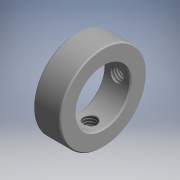
# Autodesk Inventor part: SCCJ10-5_b
Saved by Autodesk Inventor 2017.3 (Build 213256000, 256)
## iProperties
Part Number: SCCJ10-5_b
Material: Generic
Catalog Web Link: www.cadenas.de
Description: SCCJ, PSCCJ, SSCCJ_body-Set Collars - Set Screw - Standard Compact Type/2-Hole Type
Vendor: MISUMI
Document SubType Name: Modeling
Designer: partserver
Manufacturer: MISUMI
Mass: 0.57877 g
Surface Area: 6.58749 cm^2
Volume: 0.57877 cm^3
Density: 1 g/cm^3
Appearance: PSOLRGB-192-192-192
Category: PARTsolutions
Company: MISUMI
Title: SCCJ10-5
Author: Cadenas PARTsolutions
Comments: Set Collars - Set Screw - Standard Compact Type/2-Hole Type
PSOL_IDENT_0: {$CADENAS_DATA\23d-libs\misumi\metric\03_set_collars\sccj\sccj.prj},186 {VTYP=3D},{NB=SCCJ10-5_b},{L
PSOL_IDENT_1: INA=SCCJ10-5},{NN=SCCJ, PSCCJ, SSCCJ_body},{DATE=30.03.2018 01:14:32},{GEOMDATE=30.10.2015 03:01:03}
PSOL_IDENT_2: ,{VERSION=},{LINEID=40},{WBVAR=MAT,ST,BS},{WBNUMERIC=BS}  {NB=SCCJ10-5_b},{LINA=SCCJ10-5},{KT=DUMMY}
PSOL_IDENT_3: ,{PN=SCCJ10-5},{TYPE=SCCJ},{MAT=S45C},{MATALG=  'S45C','1045 Carbon Steel','SUS304','SUS304 Equivale
PSOL_IDENT_4: nt'    },{ST=B},{STALG=  'B','Black Oxide','ENP','Electroless Nickel Plating'           },{AC=Set Sc
PSOL_IDENT_5: rew 2 Pcs.},{D=10.0},{BS=5},{BS1=5},{D1=16},{DD1=0},{C=0.2},{SS=M3X3},{M1=3},{M2=3}
NB: SCCJ10-5_b
NN: SCCJ, PSCCJ, SSCCJ_body
NT: Set Collars - Set Screw - Standard Compact Type/2-Hole Type
NBSYN: $PN._b
LINA: SCCJ10-5
CATALOG: Misumi
PN: SCCJ10-5
MAT: 1045 Carbon Steel
ST: Black Oxide
AC: Set Screw 2 Pcs.
D: 10
BS: 5
D1: 16
C: 0.2
SS: M3X3
SUPPLIER: MISUMI
ARTICLENO: SCCJ10-5_b
BOMINFO: SCCJ10-5
CREATOR: CADENAS GmbH
Autodesk Inventor part; units mm, degrees
ref_plane "YZ Plane" through (0, 0, 0) normal (1, 0, 0) x (0, 1, 0)
ref_plane "XZ Plane" through (0, 0, 0) normal (0, 1, 0) x (-1, 0, 0)
ref_plane "XY Plane" through (0, 0, 0) normal (0, 0, 1) x (1, 0, 0)
sketch "Sketch_1" plane through (0, 0, 0) normal (0, 0, 1) x (1, 0, 0)
  line L0 (2, 0) -> (-2, 0)
  line L1 (-2.5, 5.2) -> (-2.3, 5)
  line L2 (-2.3, 5) -> (2.3, 5)
  line L3 (2.3, 5) -> (2.5, 5.2)
  line L4 (2.5, 5.2) -> (2.5, 7.8)
  line L5 (2.5, 7.8) -> (2.3, 8)
  line L6 (2.3, 8) -> (-2.3, 8)
  line L7 (-2.3, 8) -> (-2.5, 7.8)
  line L8 (-2.5, 7.8) -> (-2.5, 5.2)
  constraints: 18 end point
revolve "Revolution1" add sketch "Sketch_1" angle 360 about axis through (2, 0, 0) along (1, 0, 0)
sketch "Sketch_2" plane through (0, 0, 0) normal (0, 1, 0) x (-1, 0, 0)
  line L0 (0, 8) -> (0, 5)
  line L1 (0, 4) -> (-1.2295, 4)
  line L2 (-1.2295, 4) -> (-1.2295, 7.459)
  line L3 (-1.2295, 7.459) -> (-1.6074, 7.8369)
  line L4 (-1.6074, 7.8369) -> (-1.6074, 8.25)
  line L5 (-1.6074, 8.25) -> (0, 8.25)
  line L6 (0, 8.25) -> (0, 4)
  constraints: 14 end point
revolve "Revolution2" cut sketch "Sketch_2" angle 360 about axis through (0, 0, 8) along (0, 0, 1)
thread "Thread1" size "M3x0.5" class "6H" standard "ISO Metric profile" length 2.459
sketch "Sketch_6" plane through (0, 0, 0) normal (0, 0, 1) x (1, 0, 0)
  line L0 (0, 8) -> (0, 5)
  line L1 (0, 4) -> (-1.2295, 4)
  line L2 (-1.2295, 4) -> (-1.2295, 7.459)
  line L3 (-1.2295, 7.459) -> (-1.6074, 7.8369)
  line L4 (-1.6074, 7.8369) -> (-1.6074, 8.25)
  line L5 (-1.6074, 8.25) -> (0, 8.25)
  line L6 (0, 8.25) -> (0, 4)
  constraints: 14 end point
revolve "Revolution3" cut sketch "Sketch_6" angle 360 about axis through (0, 8, 0) along (0, 1, 0)
thread "Thread2" size "M3x0.5" class "6H" standard "ISO Metric profile" length 2.459
ref_plane "to_screw1_XY" through (0, 5, 0) normal (0, 1, 0) x (1, 0, 0)
ref_plane "to_screw1_YZ" through (0, 5, 0) normal (1, 0, 0) x (0, 0, -1)
ref_plane "to_screw1_ZX" through (0, 5, 0) normal (0, 0, -1) x (0, 1, 0)
ref_plane "to_screw2_XY" through (0, 0, 5) normal (0, 0, 1) x (1, 0, 0)
ref_plane "to_screw2_YZ" through (0, 0, 5) normal (1, 0, 0) x (0, 1, 0)
ref_plane "to_screw2_ZX" through (0, 0, 5) normal (0, 1, 0) x (0, 0, 1)
body "Solid1"
